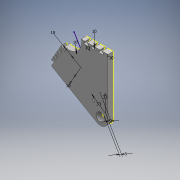
# Autodesk Inventor part: Pieza3
Saved by Autodesk Inventor 2016 (Build 200138000, 138)
## iProperties
Created: 2015-12-07
Part Number: Pieza3
Material: Genérico
Document SubType Name: Modeling
Designer: beta3
Density: 1 g/cm^3
Appearance: Valor por defecto
Author: beta3
Autodesk Inventor part; units mm, degrees
ref_plane "YZ Plane" through (0, 0, 0) normal (1, 0, 0) x (0, 1, 0)
ref_plane "XZ Plane" through (0, 0, 0) normal (0, 1, 0) x (-1, 0, 0)
ref_plane "XY Plane" through (0, 0, 0) normal (0, 0, 1) x (1, 0, 0)
sketch "Boceto1" plane through (0, 0, 0) normal (0, 1, 0) x (-1, 0, 0)
  circle A0 centre (-59.7419, -103.4763) radius 7.9656
  circle A1 centre (-47.2958, -81.9187) radius 1.9914
  line L0 (-73.6817, -103.4763) -> (-73.6817, 5.1739)
  line L1 (32.3603, -66.3972) -> (-52.772, -115.5485)
  arc A2 (-73.6817, -103.4763) -> (-52.772, -115.5485) centre (-59.7419, -103.4763) ccw
  line L2 (13.9398, -24.1443) -> (18.9183, -32.7673)
  line L3 (20.9097, -36.2166) -> (25.8882, -44.8396)
  line L4 (27.8796, -48.2888) -> (32.8581, -56.9118)
  line L5 (7.5794, -22.7716) -> (11.1559, -28.9662)
  line L6 (11.1559, -28.9662) -> (13.9398, -24.1443)
  line L7 (13.9398, -24.1443) -> (18.9183, -32.7673)
  line L8 (18.9183, -32.7673) -> (12.9441, -32.7673)
  line L9 (12.9441, -32.7673) -> (17.9226, -41.3904)
  line L10 (17.9226, -41.3904) -> (20.9097, -36.2166)
  line L11 (20.9097, -36.2166) -> (25.8882, -44.8396)
  line L12 (25.8882, -44.8396) -> (19.914, -44.8396)
  line L13 (19.914, -44.8396) -> (24.8925, -53.4626)
  line L14 (24.8925, -53.4626) -> (27.8796, -48.2888)
  line L15 (27.8796, -48.2888) -> (32.8581, -56.9118)
  line L16 (32.8581, -56.9118) -> (26.8839, -56.9118)
  line L17 (26.8839, -56.9118) -> (32.3603, -66.3972)
  line L18 (-27.8795, 0.0001) -> (-37.8365, 0.0001)
  line L19 (-41.8193, 0.0001) -> (-51.7763, 0.0001)
  line L20 (-55.7591, 0.0001) -> (-65.7161, 0.0001)
  line L21 (-23.4355, 5.1739) -> (-30.8666, 5.1739)
  line L22 (-30.8666, 5.1739) -> (-27.8795, 0.0001)
  line L23 (-27.8795, 0.0001) -> (-37.8365, 0.0001)
  line L24 (-37.8365, 0.0001) -> (-34.8494, 5.1739)
  line L25 (-34.8494, 5.1739) -> (-44.8064, 5.1739)
  line L26 (-44.8064, 5.1739) -> (-41.8193, 0.0001)
  line L27 (-41.8193, 0.0001) -> (-51.7763, 0.0001)
  line L28 (-51.7763, 0.0001) -> (-48.7892, 5.1739)
  line L29 (-48.7892, 5.1739) -> (-58.7462, 5.1739)
  line L30 (-58.7462, 5.1739) -> (-55.7591, 0.0001)
  line L31 (-55.7591, 0.0001) -> (-65.7161, 0.0001)
  line L32 (-65.7161, 0.0001) -> (-62.729, 5.1739)
  line L33 (-62.729, 5.1739) -> (-73.6817, 5.1739)
  arc A3 (-23.4355, 5.1739) -> (7.5794, -22.7716) centre (0, 0) ccw
  constraints: 68 end point, 5 collinear, 5 parallel, 4 centre point, 4 point on circle, 2 tangent, 1 coincident, 1 horizontal, 1 vertical
extrude "Extrusión2" add sketch "Boceto1" along normal blind 10
sketch "Boceto2" plane through (0, 10, 0) normal (0, 1, 0) x (1, 0, 0)
  circle A0 centre (59.7419, 103.4763) radius 7.9656 projected
  circle A1 centre (47.2958, 81.9187) radius 1.9914 projected
  arc A2 (73.6817, 103.4763) -> (52.772, 115.5485) centre (59.7419, 103.4763) ccw projected
  line L0 (52.772, 115.5485) -> (-32.3603, 66.3972) projected
  line L1 (-32.3603, 66.3972) -> (-26.8839, 56.9118) projected
  line L2 (-26.8839, 56.9118) -> (-32.8581, 56.9118) projected
  line L3 (-32.8581, 56.9118) -> (-27.8796, 48.2888) projected
  line L4 (-27.8796, 48.2888) -> (-24.8925, 53.4626) projected
  line L5 (-24.8925, 53.4626) -> (-19.914, 44.8396) projected
  line L6 (-19.914, 44.8396) -> (-25.8882, 44.8396) projected
  line L7 (-25.8882, 44.8396) -> (-20.9097, 36.2166) projected
  line L8 (-20.9097, 36.2166) -> (-17.9226, 41.3904) projected
  line L9 (-17.9226, 41.3904) -> (-12.9441, 32.7673) projected
  line L10 (-12.9441, 32.7673) -> (-18.9183, 32.7673) projected
  line L11 (-18.9183, 32.7673) -> (-13.9398, 24.1443) projected
  line L12 (-13.9398, 24.1443) -> (-11.1559, 28.9662) projected
  line L13 (-11.1559, 28.9662) -> (-7.5794, 22.7716) projected
  arc A3 (23.4355, -5.1739) -> (-7.5794, 22.7716) centre (0, 0) ccw projected
  line L14 (23.4355, -5.1739) -> (30.8666, -5.1739) projected
  line L15 (30.8666, -5.1739) -> (27.8795, -0.0001) projected
  line L16 (27.8795, -0.0001) -> (37.8365, -0.0001) projected
  line L17 (37.8365, -0.0001) -> (34.8494, -5.1739) projected
  line L18 (34.8494, -5.1739) -> (44.8064, -5.1739) projected
  line L19 (44.8064, -5.1739) -> (41.8193, -0.0001) projected
  line L20 (41.8193, -0.0001) -> (51.7763, -0.0001) projected
  line L21 (51.7763, -0.0001) -> (48.7892, -5.1739) projected
  line L22 (48.7892, -5.1739) -> (58.7462, -5.1739) projected
  line L23 (58.7462, -5.1739) -> (55.7591, -0.0001) projected
  line L24 (55.7591, -0.0001) -> (65.7161, -0.0001) projected
  line L25 (65.7161, -0.0001) -> (62.729, -5.1739) projected
  line L26 (62.729, -5.1739) -> (73.6817, -5.1739) projected
  line L27 (73.6817, -5.1739) -> (73.6817, 103.4763) projected
  line L28 (-2.0722, 33.9367) -> (-18.7001, 62.7369)
  line L29 (-18.7001, 62.7369) -> (29.3976, 90.5062)
  circle A4 centre (47.2958, 81.9187) radius 1.9914 projected
  line L30 (52.772, 115.5485) -> (-32.3603, 66.3972) projected
  arc A5 (12.4849, 31.6246) -> (-2.0722, 33.9367) centre (0, 0) ccw
  circle A6 centre (59.7419, 103.4763) radius 7.9656 projected
  arc A7 (29.3976, 90.5062) -> (39.1023, 77.7274) centre (59.7419, 103.4763) ccw
  line L31 (12.4849, 31.6246) -> (39.1023, 77.7274)
  line L32 (0, 0) -> (59.7419, 103.4763)
  line L33 (32.4961, 9.9999) -> (63.6817, 9.9999)
  line L34 (63.6817, 9.9999) -> (63.6817, 70.7123)
  line L35 (21.1452, 26.6246) -> (47.7626, 72.7274)
  arc A8 (47.7626, 72.7274) -> (63.6817, 70.7123) centre (59.7419, 103.4763) ccw
  arc A9 (32.4961, 9.9999) -> (21.1452, 26.6246) centre (0, 0) ccw
  line L36 (41.8193, -0.0001) -> (51.7763, -0.0001) projected
  line L37 (73.6817, -5.1739) -> (73.6817, 103.4763) projected
  dimension "d6" = 10
  dimension "d8" = 10
  dimension "d10" = 33
  dimension "d11" = 5
  dimension "d12" = 10
  dimension "d13" = 10
  dimension "d14" = 10
  dimension "d15" = 10
  dimension "d16" = 33
  dimension "d17" = 5
  constraints: 14 end point, 8 point on circle, 5 parallel, 4 centre point, 4 coincident, 2 perpendicular
  measures "d6" distance between parallel lines of L0 L29
  measures "d8" distance from line of L8.end L28
  measures "d10" radius of A7
  measures "d11" distance between parallel lines of L32 L31
  measures "d12" radial gap between concentric circles of A3 A5
  measures "d13" distance from line of L27 L33.end
  measures "d14" distance from line of L33 L19.end
  measures "d15" radial gap between concentric circles of A9 A3
  measures "d16" radius of A8
  measures "d17" distance from line of L32 L35.end
